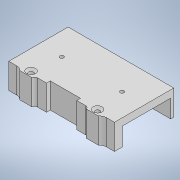
# Autodesk Inventor part: Стойка под электроннику
Saved by Autodesk Inventor 2020 (Build 240168000, 168)
## iProperties
Created: 2021-04-05
Part Number: Стойка под электроннику
Material: Типовые
Document SubType Name: Обычные детали
Designer: Антон
Density: 1 g/cm^3
Appearance: По умолчанию
Sheet Metal Rule: По умолчанию
Author: Антон
Autodesk Inventor part; units mm, degrees
ref_plane "YZ Plane" through (0, 0, 0) normal (1, 0, 0) x (0, 1, 0)
ref_plane "XZ Plane" through (0, 0, 0) normal (0, 1, 0) x (-1, 0, 0)
ref_plane "XY Plane" through (0, 0, 0) normal (0, 0, 1) x (1, 0, 0)
sketch "Эскиз1" plane through (0, 0, 0) normal (0, 1, 0) x (-1, 0, 0)
  line L0 (0, 0) -> (70, 0)
  line L1 (70, 0) -> (70, -41)
  line L2 (70, -41) -> (0, -41)
  line L3 (0, -41) -> (0, 0)
  line L4 (65, -7) -> (0, -7)
  line L5 (0, -7) -> (0, -39)
  line L6 (0, -39) -> (65, -39)
  line L7 (65, -39) -> (65, -7)
  line L8 (65, -7) -> (0, -39) construction
  line L9 (0, -7) -> (65, -39) construction
  line L10 (0, -7) -> (2, -7)
  point P0 (0, -7)
  dimension "d0" = 70
  dimension "d224" = 7
  dimension "d225" = 5
  dimension "d226" = 32
  dimension "d302" = 2
  constraints: 22 end point, 4 parallel, 3 horizontal, 2 perpendicular, 1 point on line
  measures "d0" distance of L1.end L2.end
  measures "d224" distance between parallel lines of L0 L4
  measures "d225" distance between parallel lines of L1 L7
  measures "d226" distance between parallel lines of L6 L4
  measures "d302" distance between parallel lines of L2 L6
extrude "Выдавливание1" add sketch "Эскиз1" along normal blind 12 contours L0 L1 L2 L3 L6 L7 L4
sketch "Эскиз40" plane through (0, 12, 0) normal (0, 1, 0) x (1, 0, 0)
  line L0 (0, 41) -> (-70, 41) projected
  line L1 (0, 0) -> (-70, 0)
  line L2 (-70, 0) -> (-70, 41)
  line L3 (-70, 41) -> (0, 41)
  line L4 (0, 41) -> (0, 0)
  point P0 (0, 41)
  constraints: 8 end point, 2 parallel, 1 horizontal, 1 perpendicular
extrude "Выдавливание32" add sketch "Эскиз40" along normal blind 4.8
sketch "Эскиз39" plane through (0, 16.8, 0) normal (0, 1, 0) x (1, 0, 0)
  line L0 (-70, 41) -> (-70, 0) projected
  line L1 (0, 41) -> (-70, 41) projected
  line L2 (0, 39) -> (0, 41) projected
  line L3 (-65, 39) -> (0, 39) projected
  line L4 (-65, 7) -> (-65, 39) projected
  line L5 (0, 7) -> (-65, 7) projected
  line L6 (0, 0) -> (0, 7) projected
  line L7 (-70, 0) -> (0, 0) projected
  line L8 (-70, 0) -> (0, 0) construction
  line L9 (-35, 0) -> (-35, 7) construction
  line L10 (-57.025, 3.5) -> (-12.975, 3.5) construction
  point P0 (-35, 3.5)
  dimension "d356" = 44.05
  constraints: 4 end point, 3 midpoint, 2 perpendicular, 1 point on line
  measures "d356" distance of L10.start L10.end
hole "Отверстие6" at (-12.975, 16.8, -3.5) at (-57.025, 16.8, -3.5) direction (0, -1, 0) diameter 3.2 end through all countersink diameter 6 countersink angle 90
sketch "Эскиз49" plane through (0, 12, 0) normal (0, 1, 0) x (1, 0, 0)
  line L0 (-70, 0) -> (0, 0) construction
  line L1 (-35, 0) -> (-35, 21.75) construction
  line L2 (-55, 21.75) -> (-15, 21.75) construction
  dimension "d369" = 21.75
  dimension "d370" = 40
  constraints: 4 end point, 2 midpoint, 1 horizontal, 1 perpendicular, 1 vertical
  measures "d369" distance of L1.end L1.start
  measures "d370" distance of L2.start L2.end
hole "Отверстие8" at (-15, 12, -21.75) at (-55, 12, -21.75) direction (0, 1, 0) diameter 2.5 end through all counterbore diameter 5.2 counterbore depth 3
sketch "Эскиз48" plane through (0, 16.8, 0) normal (0, 1, 0) x (1, 0, 0)
  line L0 (-53.025, 0) -> (-16.975, 0)
  line L1 (-16.975, 0) -> (-16.975, 4.2)
  line L2 (-16.975, 4.2) -> (-53.025, 4.2)
  line L3 (-53.025, 4.2) -> (-53.025, 0)
  line L4 (-70, 0) -> (0, 0) projected
  line L5 (-70, 41) -> (-70, 0) projected
  line L6 (-70, 0) -> (-61.025, 0)
  line L7 (-61.025, 0) -> (-61.025, 1.7)
  line L8 (-61.025, 1.7) -> (-70, 1.7)
  line L9 (-70, 1.7) -> (-70, 0)
  line L10 (0, 0) -> (-8.975, 0)
  line L11 (-8.975, 0) -> (-8.975, 1.7)
  line L12 (-8.975, 1.7) -> (0, 1.7)
  line L13 (0, 1.7) -> (0, 0)
  line L14 (-61.025, 0) -> (-53.025, 0)
  line L15 (-53.025, 0) -> (-53.025, 7)
  line L16 (-53.025, 7) -> (-61.025, 7)
  line L17 (-61.025, 7) -> (-61.025, 0)
  circle A0 centre (-57.025, 3.5) radius 1.6 projected
  line L18 (-61.025, 0) -> (-53.025, 7) construction
  line L19 (-53.025, 0) -> (-61.025, 7) construction
  line L20 (-8.975, 0) -> (-16.975, 0)
  line L21 (-16.975, 0) -> (-16.975, 7)
  line L22 (-16.975, 7) -> (-8.975, 7)
  line L23 (-8.975, 7) -> (-8.975, 0)
  circle A1 centre (-12.975, 3.5) radius 3 projected
  line L24 (-8.975, 0) -> (-16.975, 7) construction
  line L25 (-16.975, 0) -> (-8.975, 7) construction
  line L26 (-53.025, 0) -> (-45, 0)
  line L27 (-45, 0) -> (-45, 1.7)
  line L28 (-45, 1.7) -> (-53.025, 1.7)
  line L29 (-53.025, 1.7) -> (-53.025, 0)
  line L30 (-16.975, 0) -> (-25, 0)
  line L31 (-25, 0) -> (-25, 1.7)
  line L32 (-25, 1.7) -> (-16.975, 1.7)
  line L33 (-16.975, 1.7) -> (-16.975, 0)
  line L34 (-45, 1.7) -> (-45, 4.2)
  line L35 (-25, 1.7) -> (-25, 4.2)
  point P0 (-35, 0)
  point P1 (-8.975, 0)
  point P2 (-53.025, 1.7)
  point P3 (-16.975, 1.7)
  dimension "d359" = 4.2
  dimension "d363" = 8
  dimension "d364" = 8
  dimension "d365" = 1.7
  dimension "d366" = 8.025
  constraints: 68 end point, 14 parallel, 8 perpendicular, 7 horizontal, 6 midpoint, 5 equal length, 4 collinear, 2 point on line, 1 vertical
  measures "d359" distance of L2.end L0.start
  measures "d363" distance of L16.end L15.end
  measures "d364" distance of L21.end L22.end
  measures "d365" distance of L8.end L4.start
  measures "d366" distance of L27.end L28.end
extrude "Выдавливание38" cut sketch "Эскиз48" against normal through all contours L3 L28 L27 L0 | L27 L34 L2 L35 L31 L0 | L4 L5 L8 L7 | L31 L32 L1 L0 | L11 L12 L13 L4
fillet "Сопряжение2" radius 2 2 edges at (-16.975, 8.4, -1.7) (-53.025, 8.4, -1.7)
fillet "Сопряжение2" radius 4.7 2 edges at (-8.975, 8.4, -1.7) (-61.025, 8.4, -1.7)
